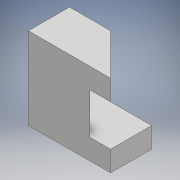
# Autodesk Inventor part: 48
Saved by Autodesk Inventor 2017 (Build 210142000, 142)
## iProperties
Part Number: 48
Material: 一般
Document SubType Name: Modeling
Designer: Brian
Density: 1 g/cm^3
Appearance: 預設
Author: Brian
Autodesk Inventor part; units mm, degrees
ref_plane "YZ Plane" through (0, 0, 0) normal (1, 0, 0) x (0, 1, 0)
ref_plane "XZ Plane" through (0, 0, 0) normal (0, 1, 0) x (-1, 0, 0)
ref_plane "XY Plane" through (0, 0, 0) normal (0, 0, 1) x (1, 0, 0)
sketch "草圖1" plane through (0, 0, 0) normal (0, 1, 0) x (-1, 0, 0)
  line L0 (0, 0) -> (-40, 0)
  line L1 (-40, 0) -> (-40, -40)
  line L2 (-40, -40) -> (0, -40)
  line L3 (0, -40) -> (0, 0)
  dimension "d0" = 40
  dimension "d1" = 40
  constraints: 8 end point, 2 parallel, 1 horizontal, 1 perpendicular
  measures "d0" distance of L2.end L0.start
  measures "d1" distance of L1.end L2.end
extrude "擠出1" add sketch "草圖1" along normal blind 20
sketch "草圖2" plane through (0, 0, 0) normal (0, 0, 1) x (1, 0, 0)
  line L0 (0, 0) -> (40, 0) projected
  line L1 (40, 0) -> (20, 20)
  line L2 (0, 20) -> (40, 20) projected
  line L3 (40, 0) -> (40, 20) projected
  line L4 (40, 0) -> (40, 20)
  dimension "d4" = 20
  constraints: 4 end point, 1 collinear, 1 midpoint
  measures "d4" horizontal distance of L0.end L1.end
extrude "擠出2" cut sketch "草圖2" against normal blind 30
sketch "草圖3" plane through (0, 0, -30) normal (0, 0, 1) x (1, 0, 0)
  line L0 (40, 0) -> (0, 0) projected
  line L1 (40, 0) -> (30, 0)
  line L2 (30, 0) -> (10, 20)
  line L3 (40, 20) -> (0, 20) projected
  line L4 (10, 20) -> (20, 20)
  line L5 (20, 20) -> (40, 0)
  dimension "d7" = 20
  dimension "d8" = 10
  constraints: 8 end point, 2 point on line, 1 midpoint
  measures "d7" horizontal distance of L1.end L2.end
  measures "d8" distance of L4.end L2.end
extrude "擠出3" cut sketch "草圖3" along normal blind 20
